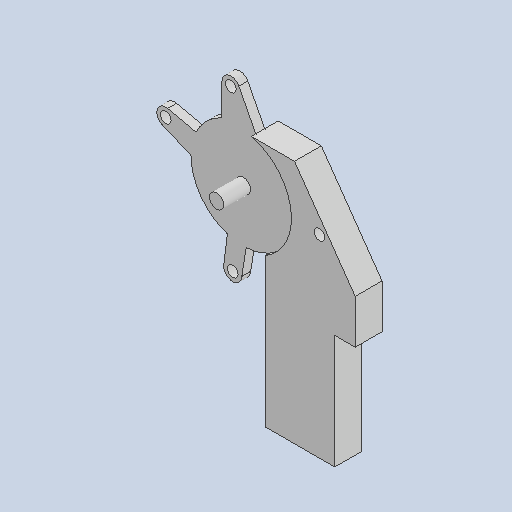
# Autodesk Inventor part: Motor
Saved by Autodesk Inventor 2025.3 (Build 293356030, 356C)
## iProperties
Created: 2026-02-08
Part Number: Motor
Material: Genérico
Document SubType Name: Modeling
Designer: Rubens
Density: 1 g/cm^3
Appearance: Padrão
Author: Rubens
Autodesk Inventor part; units mm, degrees
ref_plane "YZ Plane" through (0, 0, 0) normal (1, 0, 0) x (0, 1, 0)
ref_plane "XZ Plane" through (0, 0, 0) normal (0, 1, 0) x (-1, 0, 0)
ref_plane "XY Plane" through (0, 0, 0) normal (0, 0, 1) x (1, 0, 0)
sketch "Esboço1" plane through (0, 0, 0) normal (0, 0, 1) x (1, 0, 0)
  circle A0 centre (0, 0) radius 4
  circle A1 centre (-7, 44.6) radius 3
  circle A2 centre (45, 0) radius 3
  circle A3 centre (-6, -44.6) radius 3
  circle A4 centre (-43.5, 11.3) radius 3
  circle A5 centre (0, 0) radius 29.3573
  circle A6 centre (-7, 44.6) radius 5
  circle A7 centre (-43.5, 11.3) radius 5
  circle A8 centre (-6, -44.6) radius 5
  circle A9 centre (45, 0) radius 5
  line L0 (-12, 44.6) -> (-12, 26.7927)
  line L1 (40.0933, -0.9613) -> (42.8631, -4.0842)
  line L2 (-2.5586, 46.8966) -> (6.9412, 28.5249)
  line L3 (-45.4208, 6.6836) -> (-29.3573, 0)
  line L4 (-42.4056, 16.1788) -> (-26.5097, 12.6129)
  line L5 (-9, -27.9437) -> (-10.963, -43.993)
  line L6 (1.5707, -29.3152) -> (-1.4137, -47.5322)
  line L7 (14.7039, 28.5249) -> (31.099, 28.5249)
  line L8 (31.099, 28.5249) -> (53.6238, -3.5874)
  line L9 (-48.496, 11.5007) -> (-48.496, 11.0993)
  line L10 (14.6238, -44.6) -> (14.6238, -108.4)
  line L11 (53.6238, -44.6) -> (53.6238, -108.4)
  line L12 (53.6238, -108.4) -> (14.6238, -108.4)
  line L13 (65.104, -44.6) -> (65.104, -19.9542)
  line L14 (65.104, -19.9542) -> (49.0934, 2.8713)
  line L15 (14.6238, -44.6) -> (14.6238, -25.4557)
  line L16 (-6, -44.6) -> (-0.9333, -44.6)
  line L17 (14.6238, -44.6) -> (65.104, -44.6)
  line L18 (14.7039, 28.5249) -> (6.9412, 28.5249)
  point P0 (-1, -44.6)
  dimension "d15" = 10
  dimension "d0" = 8
  dimension "d1" = 44.6
  dimension "d2" = 7
  dimension "d3" = 6
  dimension "d4" = 6
  dimension "d5" = 45
  dimension "d6" = 6
  dimension "d7" = 44.6
  dimension "d8" = 6
  dimension "d9" = 11.3
  dimension "d10" = 6
  dimension "d11" = 37.5
  dimension "d12" = 44.6
  dimension "d13" = 10
  dimension "d14" = 10
  dimension "d16" = 10
  dimension "d17" = 0
  constraints: 38 end point, 8 centre point, 8 point on circle, 6 coincident, 6 tangent, 5 horizontal, 4 point on line, 4 vertical, 1 perpendicular, 16 other
  measures "d0" diameter of A0
  measures "d1" vertical distance of point (0, 0) A1.centre
  measures "d2" horizontal distance of point (0, 0) A1.centre
  measures "d3" diameter of A1
  measures "d4" diameter of A2
  measures "d5" distance of point (0, 0) A2.centre
  measures "d6" diameter of A3
  measures "d7" vertical distance of point (0, 0) A3.centre
  measures "d8" diameter of A4
  measures "d9" vertical distance of A0.centre A4.centre
  measures "d10" horizontal distance of A0.centre A3.centre
  measures "d11" horizontal distance of A3.centre A4.centre
  measures "d12" vertical distance of A3.centre A2.centre
  measures "d13" diameter of A6
  measures "d14" diameter of A7
  measures "d16" diameter of A9
  measures "d17" distance from line of L2.end L7
extrude "Extrusão1" add sketch "Esboço1" along normal blind 20 contours A0
extrude "Extrusão2" add sketch "Esboço1" along normal blind 5 contours A8 | A8 L5 A5 L6 L16 | A5 | L3 A7 L4 A5 | A7 L9 | L0 A6 L2 A5 | A6 picked at (-39.2458, 10.6554)
extrude "Extrusão3" add sketch "Esboço1" along normal mid plane 15 contours A9 | A5 L18 L7 L8 L14 L13 L17 L15 | L17 L11 L12 L10
